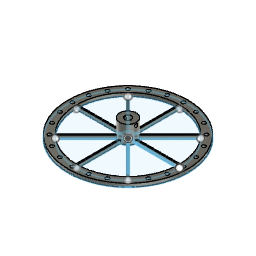
Reaction Wheel v1 (Autodesk Fusion 360 design; units mm, degrees)
Autodesk Fusion 360 part; units mm, degrees
sketch "Sketch1" plane through (0, 0, 0) normal (0, 0, 1) x (1, 0, 0)
  line L0 (-1, 0) -> (-1, -77.5)
  line L1 (-0.4142, -1) -> (77.5, -1)
  line L2 (-1, 0) -> (-1, 77.5)
  line L3 (-0.4142, 1) -> (-55.5079, -54.0937)
  line L4 (0, 0) -> (77.5, 0) construction
  line L5 (0, 0) -> (0, 77.5) construction
  line L6 (0, 0) -> (-54.8008, -54.8008) construction
  line L7 (-2.4142, 1) -> (54.0937, -55.5079)
  line L8 (0, 0) -> (0, -77.5) construction
  line L9 (-0.4142, -1) -> (-55.5079, 54.0937)
  line L10 (0, -1) -> (-77.5, -1)
  line L11 (2.4142, 1) -> (55.5079, 54.0937)
  line L12 (0, 0) -> (77.5, 0) construction
  line L13 (0.7071, 0.7071) -> (-54.0937, 55.5079)
  line L14 (0, 0) -> (-54.8008, 54.8008) construction
  line L15 (2.4142, 1) -> (77.5, 1)
  line L16 (0, 1) -> (-77.5, 1)
  circle A0 centre (0, 0) radius 12.5
  line L17 (-2.4142, 1) -> (77.5, 1)
  line L18 (-0.4142, 1) -> (77.5, 1)
  line L19 (2.4142, -1) -> (77.5, -1)
  line L20 (-2.4142, -1) -> (77.5, -1)
  line L21 (0, 0) -> (-77.5, 0) construction
  circle A1 centre (0, 0) radius 5.05
  line L22 (1, 0) -> (1, -77.5)
  line L23 (0.4142, -1) -> (-54.0937, -55.5079)
  line L24 (0, 0) -> (54.8008, 54.8008) construction
  line L25 (1, 0) -> (1, 77.5)
  line L26 (0, 0) -> (77.5, 0) construction
  circle A2 centre (0, 0) radius 77.5
  line L27 (0, 0) -> (77.5, 0) construction
  circle A3 centre (0, 0) radius 90
  line L28 (0.4142, -1) -> (77.5, -1)
  line L29 (0, 0) -> (54.8008, -54.8008) construction
  line L30 (-2.4142, -1) -> (54.0937, 55.5079)
  line L31 (0, 0) -> (77.5, 0) construction
  line L32 (2.4142, -1) -> (55.5079, -54.0937)
  dimension "d42" = 1
  dimension "d43" = -1
  dimension "d44" = 1
  dimension "d45" = -1
  dimension "d46" = 1
  dimension "d47" = -1
  dimension "d48" = 1
  dimension "d49" = -1
  dimension "d50" = 1
  dimension "d51" = -1
  dimension "d52" = 1
  dimension "d53" = -1
  dimension "d54" = 1
  dimension "d55" = -1
  dimension "d33" = 10.1
  dimension "d35" = 180
  dimension "d37" = 155
  dimension "d38" = 45
  dimension "d39" = 45
  dimension "d40" = 135
  dimension "d41" = 135
  dimension "d56" = 25
  constraint coincident L4.start L5.start
  constraint concentric A1 A3
  constraint concentric A1 A2
  constraint coincident L21.end A2
  constraint horizontal L21
  constraint coincident L5.end A2
  constraint perpendicular L5 L21
  constraint coincident L4.end A2
  constraint perpendicular L5 L27
  constraint coincident L8.end A2
  constraint perpendicular L8 L27
  constraint horizontal L12
  constraint horizontal L26
  constraint horizontal L4
  constraint horizontal L31
  constraint concentric A0 A1
  measures "d33" diameter of A1
  measures "d35" diameter of A3
  measures "d37" diameter of A2
  measures "d38" angle of L12 L24
  measures "d39" angle of L26 L29
  measures "d40" angle of L4 L14
  measures "d41" angle of L6 L31
  measures "d56" diameter of A0
extrude "Extrude1" add sketch "Sketch1" along normal blind 27 contours L0 A0 A1 L22 | L0 A0 A1 L23 | L3 A0 A1 L23 | L3 L10 A0 A1 | L10 L16 A0 A1 | L9 L16 A0 A1 | L9 L13 A0 A1 | L2 L13 A0 A1 | L2 A0 A1 L25 | L7 A0 A1 L22 | L7 A0 A1 L32 | A0 A1 L25 L30 | L11 A0 A1 L30 | L1 A0 L19 L20 A1 L28 L32 | L11 L15 A0 L17 L18 A1 | L1 L15 A0 L17 L18 L19 L20 A1 L28
extrude "Extrude2" add sketch "Sketch1" along normal blind 5 contours L0 A0 L22 A2 | L3 A0 L23 A2 | L10 L16 A0 A2 | L9 L13 A0 A2 | L2 A0 L25 A2 | L7 A0 A2 L32 | L11 A0 A2 L30 | L1 L15 A0 L17 L18 L19 L20 A2 L28 | A3
sketch "Sketch2" plane through (0, 0, 5) normal (0, 0, 1) x (-1, 0, 0)
  arc A0 (1, 12.4599) -> (-1, 12.4599) centre (0, 0) ccw
  line L0 (1, 12.4599) -> (1, 77.4935)
  arc A1 (54.0891, 55.5033) -> (1, 77.4935) centre (0, 0) ccw
  line L1 (54.0891, 55.5033) -> (8.1034, 9.5176)
  arc A2 (9.5176, 8.1034) -> (8.1034, 9.5176) centre (0, 0) ccw
  line L2 (9.5176, 8.1034) -> (55.5033, 54.0891)
  arc A3 (77.4935, 1) -> (55.5033, 54.0891) centre (0, 0) ccw
  line L3 (77.4935, 1) -> (12.4599, 1)
  arc A4 (12.4599, -1) -> (12.4599, 1) centre (0, 0) ccw
  line L4 (12.4599, -1) -> (77.4935, -1)
  arc A5 (55.5033, -54.0891) -> (77.4935, -1) centre (0, 0) ccw
  line L5 (55.5033, -54.0891) -> (9.5176, -8.1034)
  arc A6 (8.1034, -9.5176) -> (9.5176, -8.1034) centre (0, 0) ccw
  line L6 (8.1034, -9.5176) -> (54.0891, -55.5033)
  arc A7 (1, -77.4935) -> (54.0891, -55.5033) centre (0, 0) ccw
  line L7 (1, -77.4935) -> (1, -12.4599)
  arc A8 (-1, -12.4599) -> (1, -12.4599) centre (0, 0) ccw
  line L8 (-1, -12.4599) -> (-1, -77.4935)
  arc A9 (-54.0891, -55.5033) -> (-1, -77.4935) centre (0, 0) ccw
  line L9 (-54.0891, -55.5033) -> (-8.1034, -9.5176)
  arc A10 (-9.5176, -8.1034) -> (-8.1034, -9.5176) centre (0, 0) ccw
  line L10 (-9.5176, -8.1034) -> (-55.5033, -54.0891)
  arc A11 (-77.4935, -1) -> (-55.5033, -54.0891) centre (0, 0) ccw
  line L11 (-77.4935, -1) -> (-12.4599, -1)
  arc A12 (-12.4599, 1) -> (-12.4599, -1) centre (0, 0) ccw
  line L12 (-12.4599, 1) -> (-77.4935, 1)
  arc A13 (-55.5033, 54.0891) -> (-77.4935, 1) centre (0, 0) ccw
  line L13 (-55.5033, 54.0891) -> (-9.5176, 8.1034)
  arc A14 (-8.1034, 9.5176) -> (-9.5176, 8.1034) centre (0, 0) ccw
  line L14 (-8.1034, 9.5176) -> (-54.0891, 55.5033)
  arc A15 (-1, 77.4935) -> (-54.0891, 55.5033) centre (0, 0) ccw
  line L15 (-1, 77.4935) -> (-1, 12.4599)
  circle A16 centre (0, 0) radius 90
  line L16 (-77.5, 0) -> (-83.75, 0) construction
  circle A17 centre (-83.75, 0) radius 2.65
  point P0 (-77.5, 0)
  dimension "d28" = 6.25
  dimension "d29" = 5.3
  constraint coincident P0 L16.start
  constraint horizontal L16
  constraint coincident L16.end A17.centre
  measures "d28" distance of P0 L16.end
  measures "d29" diameter of A17
hole "Hole1" at (83.75, 0, 5) direction (0, 0, -1) diameter 5.3 depth 10 tip angle 180
pattern_circular "C-Pattern1" count 24 over 360 about axis through (0, 0, 0) along (0, 0, 1) of "Hole1"
ref_plane "WorkPlane1" through (12.5, 0, 19.1773) normal (1, 0, 0) x (0, -1, 0)
ref_plane "WorkPlane2" through (-12.5, 0, 14.5915) normal (-1, 0, 0) x (0, 1, 0)
ref_plane "WorkPlane3" through (0, 0, 14.5915) normal (-1, 0, 0) x (0, 1, 0)
sketch "Sketch3" plane through (0, 0, 14.5915) normal (-1, 0, 0) x (0, 1, 0)
  line L0 (-12.5, -12.4085) -> (12.5, -12.4085)
  line L1 (0, -12.4085) -> (0, -8.4085)
  circle A0 centre (0, -8.4085) radius 2.5
  dimension "d59" = 4
  dimension "d60" = 5
  constraint midpoint L0 L1.start
  constraint perpendicular L0 L1
  constraint coincident L1.end A0.centre
  measures "d59" distance of L1.start L1.end
  measures "d60" diameter of A0
extrude "Extrude3" cut sketch "Sketch3" along normal blind 16 and the other way blind 18
equation "d28 = ( 12.500 / 2 ) * 1 mm"
